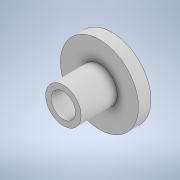
# Autodesk Inventor part: 017
Saved by Autodesk Inventor 2022.2 (Build 262287000, 287)
## iProperties
Manager: Angie Guevara
Company: ITM
Created: 2021-11-08
Part Number: 017
Material: Genérico
Document SubType Name: Modeling
Designer: Samuel Gómez
Density: 1 g/cm^3
Appearance: Valor por defecto
Checked By: Angie Guevara
Engr Approved By: Angie Guevara
Engineer: Angie Guevara
Author: Samuel Gómez
Autodesk Inventor part; units mm, degrees
ref_plane "YZ Plane" through (0, 0, 0) normal (1, 0, 0) x (0, 1, 0)
ref_plane "XZ Plane" through (0, 0, 0) normal (0, 1, 0) x (-1, 0, 0)
sketch "Boceto1" plane through (0, 0, 0) normal (0, 0, 1) x (1, 0, 0)
  circle A0 centre (0, 0) radius 4.98
  circle A1 centre (0, 0) radius 3.425
  constraints: 2 centre point, 2 coincident
extrude "Extrusión1" add sketch "Boceto1" along normal blind 15
ref_plane "Plano de trabajo1" through (0, 0, 4.83) normal (0, 0, 1) x (1, 0, 0)
sketch "Boceto2" plane through (0, 0, 4.83) normal (0, 0, 1) x (1, 0, 0)
  circle A0 centre (0, 0) radius 10.975
  circle A1 centre (0, 0) radius 4.98
  dimension "d5" = 21.95
  constraints: 2 centre point, 2 coincident
  measures "d5" diameter of A0
extrude "Extrusión2" add sketch "Boceto2" against normal blind 3.5
